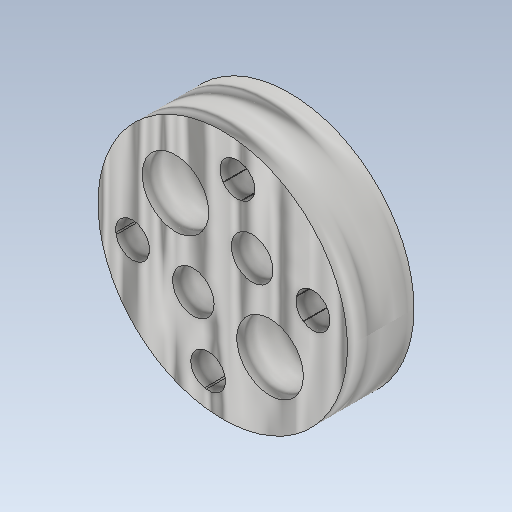
# Autodesk Inventor part: 新型３脚カム
Saved by Autodesk Inventor 2020 (Build 240168000, 168)
## iProperties
Created: 2019-04-15
Part Number: 新型３脚カム
Material: アルミニウム 7075
Document SubType Name: Modeling
Designer: tanjihayato
Density: 2.81 g/cm^3
Appearance: サテン - ブラシ仕上げ 重厚
Mass: 1.44307 g
Surface Area: 7.12387 cm^2
Volume: 0.513548 cm^3
Author: tanjihayato
Autodesk Inventor part; units mm, degrees
ref_plane "YZ Plane" through (0, 0, 0) normal (1, 0, 0) x (0, 1, 0)
ref_plane "XZ Plane" through (0, 0, 0) normal (0, 1, 0) x (-1, 0, 0)
ref_plane "XY Plane" through (0, 0, 0) normal (0, 0, 1) x (1, 0, 0)
sketch "スケッチ1" plane through (0, 0, 0) normal (0, 0, 1) x (1, 0, 0)
  circle A0 centre (-12.0208, 12.0208) radius 9.5
  arc A1 (-18.7383, 18.7383) -> (-18.7383, -18.7383) centre (0, 0) ccw
  circle A2 centre (-14.8669, 14.8669) radius 2
  circle A3 centre (-10.253, 13.7886) radius 1.25
  circle A4 centre (-13.7886, 10.253) radius 1.25
  circle A5 centre (-9.1747, 9.1747) radius 2
  circle A6 centre (-12.0208, -12.0208) radius 9.5
  arc A7 (-8.2499, -13.092) -> (-13.092, -8.2499) centre (-9.1747, -9.1747) ccw
  circle A8 centre (-9.1747, -9.1747) radius 2
  circle A9 centre (-13.7886, -10.253) radius 1.25
  arc A10 (-13.9423, -9.0125) -> (-13.092, -8.2499) centre (-14.0653, -8.0201) ccw
  arc A11 (-15.7917, -10.9496) -> (-15.0291, -10.0993) centre (-16.0215, -9.9764) ccw
  arc A12 (-15.7917, -10.9496) -> (-10.9496, -15.7917) centre (-14.8669, -14.8669) ccw
  circle A13 centre (-14.8669, -14.8669) radius 2
  circle A14 centre (-10.253, -13.7886) radius 1.25
  arc A15 (-10.0993, -15.0291) -> (-10.9496, -15.7917) centre (-9.9764, -16.0215) ccw
  arc A16 (-10.0993, -15.0291) -> (-9.0125, -13.9423) centre (-10.253, -13.7886) ccw
  arc A17 (-8.2499, -13.092) -> (-9.0125, -13.9423) centre (-8.0201, -14.0653) ccw
  arc A18 (-7.6297, -14.4272) -> (-14.4272, -7.6297) centre (-9.1747, -9.1747) ccw
  arc A19 (-9.6145, -16.412) -> (-7.6297, -14.4272) centre (-10.253, -13.7886) ccw
  arc A20 (-16.412, -9.6145) -> (-9.6145, -16.412) centre (-14.8669, -14.8669) ccw
  arc A21 (-14.4272, -7.6297) -> (-16.412, -9.6145) centre (-13.7886, -10.253) ccw
  arc A22 (-11.6204, 16.1746) -> (-16.1746, 11.6204) centre (-14.8669, 14.8669) ccw
  arc A23 (-7.8671, 12.4213) -> (-11.6204, 16.1746) centre (-10.253, 13.7886) ccw
  arc A24 (-16.1746, 11.6204) -> (-12.4213, 7.8671) centre (-13.7886, 10.253) ccw
  arc A25 (-12.4213, 7.8671) -> (-7.8671, 12.4213) centre (-9.1747, 9.1747) ccw
  circle A26 centre (-12.0208, -12.0208) radius 8
  line L0 (-25.4165, 7.5) -> (-25.4165, -7.5)
  line L1 (-23.9165, 7.2801) -> (-23.9165, -7.2801)
  arc A27 (-21.491, 12.7724) -> (-23.9165, 7.2801) centre (0, 0) ccw
  arc A28 (-23.9165, -7.2801) -> (-21.491, -12.7724) centre (0, 0) ccw
  line L2 (-2.5208, 12.0208) -> (-2.5208, -12.0208)
  line L3 (-4.0208, 6.8973) -> (-4.0208, -6.8973)
  circle A29 centre (-12.0208, 12.0208) radius 7.5
  line L4 (-13.7886, -10.253) -> (-4.0461, -19.9955) construction
  line L5 (-13.7886, 10.253) -> (-4.0869, 19.9547) construction
  line L6 (-12.7708, 2.5505) -> (-12.7708, -2.5505)
  line L7 (-11.2708, 2.5505) -> (-11.2708, -2.5505)
  arc A30 (-10.8714, 16.4682) -> (-10.9282, 18.4283) centre (-11.0963, 17.4426) ccw
  arc A31 (-5.6133, 13.1135) -> (-7.5735, 13.1702) centre (-6.5991, 12.9454) ccw
  arc A32 (-13.1702, 7.5735) -> (-13.1135, 5.6133) centre (-12.9454, 6.5991) ccw
  arc A33 (-18.4283, 10.9282) -> (-16.4682, 10.8714) centre (-17.4426, 11.0963) ccw
  arc A34 (-10.9282, 18.4283) -> (-13.9213, 18.2368) centre (-12.0208, 12.0208) ccw
  arc A35 (-18.2368, 13.9213) -> (-18.4283, 10.9282) centre (-12.0208, 12.0208) ccw
  arc A36 (-13.1135, 5.6133) -> (-10.1203, 5.8049) centre (-12.0208, 12.0208) ccw
  arc A37 (-5.8049, 10.1203) -> (-5.6133, 13.1135) centre (-12.0208, 12.0208) ccw
  point P0 (0, 0)
  point P1 (0, 0)
  point P2 (-5.3033, -18.7383)
  point P3 (-5.3033, 18.7383)
  dimension "d0" = 1.45
  dimension "d1" = 1.45
  dimension "d2" = 1.5
  dimension "d3" = 1.5
  dimension "d4" = 1.5
  dimension "d5" = 1.5
  dimension "d6" = 1.5
  dimension "d7" = 15
  dimension "d8" = 1.5
  dimension "d9" = 1.5
  dimension "d10" = 1.5
  dimension "d11" = 1.5
  dimension "d12" = 15
  dimension "d13" = 1.5
  dimension "d14" = 0.75
  dimension "d16" = 2
  dimension "d17" = 2
  dimension "d18" = 2
  dimension "d19" = 2
  dimension "d23" = 4
  dimension "d24" = 4
  dimension "d25" = 1
  dimension "d26" = 1
  dimension "d27" = 1
  dimension "d28" = 1
  constraints: 62 point on circle, 36 centre point, 16 end point, 8 tangent, 6 vertical, 2 point on line, 1 coincident, 1 parallel, 20 other
  measures "d0" radial gap between concentric circles of A16 A19
  measures "d1" radial gap between concentric circles of A9 A21
  measures "d2" radial gap between concentric circles of A3 A23
  measures "d3" radial gap between concentric circles of A2 A22
  measures "d4" radial gap between concentric circles of A24 A4
  measures "d5" radial gap between concentric circles of A25 A5
  measures "d7" distance of L0.start L0.end
  measures "d8" distance between parallel lines of L1 L0
  measures "d9" radial gap between concentric circles of A1 A27
  measures "d10" radial gap between concentric circles of A1 A28
  measures "d11" distance between parallel lines of L3 L2
  measures "d12" diameter of A29
  measures "d13" distance between parallel lines of L6 L7
  measures "d14" distance from line of point (-12.021, 12.021) L7
  measures "d16" diameter of A30
  measures "d17" diameter of A31
  measures "d18" diameter of A32
  measures "d19" diameter of A33
  measures "d23" diameter of A2
  measures "d24" diameter of A5
  measures "d25" radial gap between concentric circles of A29 A35
  measures "d26" radial gap between concentric circles of A29 A36
  measures "d27" radial gap between concentric circles of A29 A37
  measures "d28" radial gap between concentric circles of A29 A34
extrude "押し出し1" add sketch "スケッチ1" along normal blind 4 contours A23 A25 A29 A24 A22 | A22 A29 A25 A37 A31 A23 A30 A34 | A22 A35 A33 A24 A32 A36 A25 A29
fillet "フィレット1" radius 1 8 edges at (-10.1203, 5.8049, 2) (-12.4213, 7.8671, 2) (-16.1746, 11.6204, 2) (-18.2368, 13.9213, 2) (-7.8671, 12.4213, 2) (-5.8049, 10.1203, 2) (-13.9213, 18.2368, 2) (-11.6204, 16.1746, 2)
